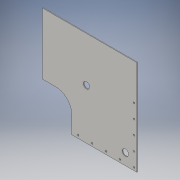
# Autodesk Inventor part: 1073-2017 Shooter Outside Plate Left
Saved by Autodesk Inventor 2016 (Build 200138000, 138)
## iProperties
Created: 2017-01-29
Part Number: 1073-2017 Shooter Outside Plate Left
Material: Generic
Document SubType Name: Modeling
Designer: rasmussenf
Density: 1 g/cm^3
Appearance: Default
Author: rasmussenf
Autodesk Inventor part; units mm, degrees
ref_plane "YZ Plane" through (0, 0, 0) normal (1, 0, 0) x (0, 1, 0)
ref_plane "XZ Plane" through (0, 0, 0) normal (0, 1, 0) x (-1, 0, 0)
ref_plane "XY Plane" through (0, 0, 0) normal (0, 0, 1) x (1, 0, 0)
sketch "Sketch1" plane through (0, 0, 0) normal (0, 0, 1) x (1, 0, 0)
  line L0 (133.35, 0) -> (428.625, 0)
  line L1 (428.625, 0) -> (428.625, 431.8)
  line L2 (428.625, 431.8) -> (0, 431.8)
  circle A0 centre (200.025, 228.6) radius 14.2875
  circle A1 centre (200.025, 228.6) radius 250.0376 construction
  circle A2 centre (376.8283, 51.7967) radius 14.2875
  line L3 (200.025, 228.6) -> (428.625, 0) construction
  line L4 (0, 152.4) -> (60.325, 152.4)
  line L5 (133.35, 79.375) -> (133.35, 0)
  arc A3 (133.35, 79.375) -> (60.325, 152.4) centre (60.325, 79.375) ccw
  line L6 (0, 431.8) -> (0, 152.4)
  point P0 (0, 0)
  dimension "d5" = 500.0752
  dimension "d0" = 428.625
  dimension "d1" = 431.8
  dimension "d2" = 28.575
  dimension "d3" = 228.6
  dimension "d4" = 228.6
  dimension "d6" = 28.575
  dimension "d7" = 152.4
  dimension "d8" = 295.275
  dimension "d9" = 73.025
  constraints: 14 end point, 3 centre point, 2 horizontal, 2 parallel, 2 perpendicular, 2 point on circle, 2 tangent, 1 coincident, 1 point on line, 3 other
  measures "d0" distance of L1.end L2.end
  measures "d1" distance of L0.end L1.end
  measures "d2" diameter of A0
  measures "d3" distance from line of L1 A0.centre
  measures "d4" distance from line of L0 A0.centre
  measures "d6" diameter of A2
  measures "d7" distance from line of L0 L4.start
  measures "d8" distance from line of L0.start L1
  measures "d9" radius of A3
extrude "Extrusion1" add sketch "Sketch1" along normal blind 3.175
sketch "Sketch2" plane through (0, 0, 3.175) normal (0, 0, 1) x (1, 0, 0)
  circle A0 centre (415.925, 12.7) radius 3.5687
  line L0 (133.35, 0) -> (428.625, 0) projected
  line L1 (428.625, 0) -> (428.625, 431.8) projected
  circle A1 centre (415.925, 76.2) radius 3.5687
  circle A2 centre (415.925, 139.7) radius 3.5687
  circle A3 centre (415.925, 203.2) radius 3.5687
  circle A4 centre (415.925, 266.7) radius 3.5687
  circle A5 centre (352.425, 12.7) radius 3.5687
  circle A6 centre (288.925, 12.7) radius 3.5687
  circle A7 centre (225.425, 12.7) radius 3.5687
  circle A8 centre (161.925, 12.7) radius 3.5687
  point P0 (0, 0)
  dimension "d12" = 7.1374
  dimension "d13" = 12.7
  dimension "d14" = 12.7
  dimension "d17" = 63.5
  dimension "d27" = 63.5
  constraints: 9 centre point, 1 horizontal, 1 vertical, 16 other
  measures "d12" diameter of A0
  measures "d13" distance from line of L0 A0.centre
  measures "d14" distance from line of L1 A0.centre
  measures "d17" distance of A0.centre A1.centre
  measures "d27" distance of A0.centre A5.centre
extrude "Extrusion2" cut sketch "Sketch2" against normal blind 3.175
body "Solid1"
